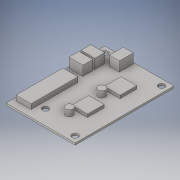
# Autodesk Inventor part: PCB
Saved by Autodesk Inventor 2016 (Build 200138000, 138)
## iProperties
Created: 2015-09-25
Part Number: PCB
Material: Generic
Document SubType Name: Modeling
Designer: lachesis
Density: 1 g/cm^3
Appearance: Default
Author: lachesis
Autodesk Inventor part; units mm, degrees
ref_plane "YZ Plane" through (0, 0, 0) normal (1, 0, 0) x (0, 1, 0)
ref_plane "XZ Plane" through (0, 0, 0) normal (0, 1, 0) x (-1, 0, 0)
ref_plane "XY Plane" through (0, 0, 0) normal (0, 0, 1) x (1, 0, 0)
sketch "Sketch1" plane through (0, 0, 0) normal (0, 1, 0) x (-1, 0, 0)
  line L0 (35.56, 50.8) -> (-35.56, 50.8)
  line L1 (-35.56, 50.8) -> (-35.56, -50.8)
  line L2 (-35.56, -50.8) -> (35.56, -50.8)
  line L3 (35.56, -50.8) -> (35.56, 50.8)
  point P0 (0, 0)
  point P1 (35.56, 0)
  point P2 (0, -50.8)
  dimension "d0" = 101.6
  dimension "d1" = 71.12
  constraints: 8 end point, 2 midpoint, 2 parallel, 1 horizontal, 1 horizontal alignment, 1 perpendicular, 1 vertical alignment
  measures "d0" distance of L2.end L0.start
  measures "d1" distance of L1.end L2.end
extrude "Extrusion1" add sketch "Sketch1" along normal blind 2
sketch "Sketch2" plane through (0, 2, 0) normal (0, 1, 0) x (1, 0, 0)
  line L0 (-35.56, 50.8) -> (-35.56, -50.8) projected
  line L1 (35.56, 50.8) -> (-35.56, 50.8) projected
  line L2 (35.56, -50.8) -> (35.56, 50.8) projected
  line L3 (-35.56, -50.8) -> (35.56, -50.8) projected
  point P0 (0, 0)
  point P1 (-10.16, -35.56)
  point P2 (-29.21, 44.45)
  point P3 (29.21, 44.45)
  point P4 (29.21, -44.45)
  dimension "d4" = 6.35
  dimension "d5" = 6.35
  dimension "d6" = 6.35
  dimension "d7" = 6.35
  dimension "d8" = 15.24
  dimension "d9" = 45.72
  constraints: 1 horizontal alignment, 1 vertical alignment
  measures "d4" distance from line of L0 point (-29.21, 44.45)
  measures "d5" distance from line of L1 point (-29.21, 44.45)
  measures "d6" distance from line of L2 point (29.21, 44.45)
  measures "d7" distance from line of point (29.21, -44.45) L3
  measures "d8" vertical distance of L2.start point (-10.16, -35.56)
  measures "d9" horizontal distance of L2.start point (-10.16, -35.56)
hole "Hole1" at (-10.16, 2, 35.56) at (-29.21, 2, -44.45) at (29.21, 2, -44.45) at (29.21, 2, 44.45) direction (0, -1, 0) diameter 6.35 end through all
sketch "Sketch3" plane through (0, 2, 0) normal (0, 1, 0) x (1, 0, 0)
  line L0 (-32.412, -43.7017) -> (-16.972, -43.7017)
  line L1 (-16.972, -43.7017) -> (-16.972, 4.5583)
  line L2 (-16.972, 4.5583) -> (-32.412, 4.5583)
  line L3 (-32.412, 4.5583) -> (-32.412, -43.7017)
  line L4 (-35.56, -50.8) -> (35.56, -50.8) projected
  line L5 (-35.56, 50.8) -> (-35.56, -50.8) projected
  point P0 (0, 0)
  dimension "d17" = 15.44
  dimension "d18" = 48.26
  dimension "d19" = 7.0983
  dimension "d20" = 3.148
  constraints: 8 end point, 2 parallel, 1 perpendicular
  measures "d17" distance of L1.end L2.end
  measures "d18" distance of L2.end L0.start
  measures "d19" distance between parallel lines of L0 L4
  measures "d20" distance between parallel lines of L5 L3
extrude "Extrusion2" add sketch "Sketch3" along normal blind 5.08
sketch "Sketch4" plane through (0, 2, 0) normal (0, 1, 0) x (1, 0, 0)
  line L0 (-34.03, 12.4581) -> (-19.81, 12.4581)
  line L1 (-19.81, 12.4581) -> (-19.81, 22.6181)
  line L2 (-19.81, 22.6181) -> (-34.03, 22.6181)
  line L3 (-34.03, 22.6181) -> (-34.03, 12.4581)
  line L4 (-34.03, 24.6781) -> (-19.81, 24.6781)
  line L5 (-19.81, 24.6781) -> (-19.81, 34.8381)
  line L6 (-19.81, 34.8381) -> (-34.03, 34.8381)
  line L7 (-34.03, 34.8381) -> (-34.03, 24.6781)
  line L8 (-14.98, 35.05) -> (-4.82, 35.05)
  line L9 (-4.82, 35.05) -> (-4.82, 49.27)
  line L10 (-4.82, 49.27) -> (-14.98, 49.27)
  line L11 (-14.98, 49.27) -> (-14.98, 35.05)
  line L12 (-16.972, 4.5583) -> (-32.412, 4.5583) projected
  line L13 (-35.56, 50.8) -> (-35.56, -50.8) projected
  line L14 (35.56, 50.8) -> (-35.56, 50.8) projected
  point P0 (0, 0)
  dimension "d23" = 14.22
  dimension "d24" = 10.16
  dimension "d25" = 2.06
  dimension "d26" = 7.8999
  dimension "d27" = 1.53
  dimension "d28" = 1.53
  dimension "d29" = 20.58
  constraints: 24 end point, 6 parallel, 3 equal length, 3 horizontal, 3 perpendicular, 2 point on line
  measures "d23" distance of L0.start L0.end
  measures "d24" distance of L2.end L0.start
  measures "d25" distance between parallel lines of L4 L2
  measures "d26" distance between parallel lines of L12 L0
  measures "d27" distance between parallel lines of L13 L3
  measures "d28" distance between parallel lines of L14 L10
  measures "d29" distance between parallel lines of L13 L11
extrude "Extrusion3" add sketch "Sketch4" along normal blind 10
sketch "Sketch5" plane through (0, 2, 0) normal (0, 1, 0) x (1, 0, 0)
  line L0 (3.1628, -21.8228) -> (19.1628, -21.8228)
  line L1 (19.1628, -21.8228) -> (19.1628, -4.6228)
  line L2 (19.1628, -4.6228) -> (3.1628, -4.6228)
  line L3 (3.1628, -4.6228) -> (3.1628, -21.8228)
  line L4 (3.1628, 11.7072) -> (19.1628, 11.7072)
  line L5 (19.1628, 11.7072) -> (19.1628, 28.9072)
  line L6 (19.1628, 28.9072) -> (3.1628, 28.9072)
  line L7 (3.1628, 28.9072) -> (3.1628, 11.7072)
  line L8 (35.56, -50.8) -> (35.56, 50.8) projected
  line L9 (35.56, 50.8) -> (-35.56, 50.8) projected
  point P0 (0, 0)
  dimension "d32" = 17.2
  dimension "d33" = 16
  dimension "d34" = 16.33
  dimension "d35" = 16.3972
  dimension "d36" = 21.8928
  constraints: 16 end point, 4 parallel, 2 equal length, 2 horizontal, 2 perpendicular, 1 collinear
  measures "d32" distance of L0.end L1.end
  measures "d33" distance of L1.end L2.end
  measures "d34" distance between parallel lines of L4 L2
  measures "d35" distance between parallel lines of L8 L1
  measures "d36" distance between parallel lines of L9 L6
extrude "Extrusion4" add sketch "Sketch5" along normal blind 3
sketch "Sketch6" plane through (0, 2, 0) normal (0, 1, 0) x (1, 0, 0)
  circle A0 centre (6.61, -27.94) radius 3.75
  circle A1 centre (6.61, 5.58) radius 3.75
  line L0 (35.56, -50.8) -> (35.56, 50.8) projected
  line L1 (-35.56, -50.8) -> (35.56, -50.8) projected
  point P0 (0, 0)
  dimension "d39" = 7.5
  dimension "d40" = 26.02
  dimension "d41" = 25.2
  dimension "d42" = 19.11
  constraints: 2 centre point, 1 equal radius, 1 vertical alignment
  measures "d39" diameter of A0
  measures "d41" distance edge to line of A1 L0
  measures "d42" distance edge to line of A0 L1
extrude "Extrusion5" add sketch "Sketch6" along normal blind 6.35
equation "\"d5\" = d4"
equation "\"d6\" = d4"
equation "\"d7\" = d4"
body "Solid1"
